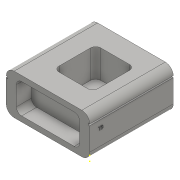
# Autodesk Inventor part: PassengerSectionNT
Saved by Autodesk Inventor 2016 (Build 200138000, 138)
## iProperties
Created: 2016-01-08
Part Number: PassengerSectionNT
Material: Generic
Document SubType Name: Modeling
Designer: 301278
Density: 1 g/cm^3
Appearance: Default
Author: 301278
Autodesk Inventor part; units mm, degrees
ref_plane "YZ Plane" through (0, 0, 0) normal (1, 0, 0) x (0, 1, 0)
ref_plane "XZ Plane" through (0, 0, 0) normal (0, 1, 0) x (-1, 0, 0)
ref_plane "XY Plane" through (0, 0, 0) normal (0, 0, 1) x (1, 0, 0)
sketch "Sketch1" plane through (0, 0, 0) normal (0, 0, 1) x (1, 0, 0)
  point P0 (0, 0)
sketch "Sketch2" plane through (0, 0, 0) normal (0, 0, 1) x (1, 0, 0)
  line L0 (7.62, 0) -> (72.898, 0)
  line L1 (80.518, 7.62) -> (80.518, 31.242)
  line L2 (72.898, 38.862) -> (7.62, 38.862)
  line L3 (0, 31.242) -> (0, 7.62)
  arc A0 (7.62, 38.862) -> (0, 31.242) centre (7.62, 31.242) ccw
  arc A1 (80.518, 31.242) -> (72.898, 38.862) centre (72.898, 31.242) ccw
  arc A2 (72.898, 0) -> (80.518, 7.62) centre (72.898, 7.62) ccw
  arc A3 (0, 7.62) -> (7.62, 0) centre (7.62, 7.62) ccw
  point P0 (0, 0)
  point P1 (80.518, 38.862)
  point P2 (80.518, 0)
  point P3 (0, 38.862)
  dimension "d0" = 80.518
  dimension "d1" = 38.862
  dimension "d2" = 7.62
  dimension "d3" = 7.62
  constraints: 8 end point, 8 point on circle, 8 point on line, 8 tangent, 4 centre point, 2 equal radius, 2 parallel, 1 horizontal, 1 perpendicular
  measures "d0" distance of point (0, 38.862) point (80.518, 38.862)
  measures "d1" distance of point (80.518, 38.862) point (80.518, 0)
  measures "d2" radius of A0
  measures "d3" radius of A1
extrude "Extrusion1" add sketch "Sketch2" along normal blind 80.518
sketch "Sketch3" plane through (0, 0, 80.518) normal (0, 0, 1) x (1, 0, 0)
  line L0 (13.716, 32.004) -> (66.802, 32.004)
  line L1 (71.882, 26.924) -> (71.882, 10.16)
  line L2 (66.802, 5.08) -> (13.716, 5.08)
  line L3 (8.636, 10.16) -> (8.636, 26.924)
  arc A0 (13.716, 32.004) -> (8.636, 26.924) centre (13.716, 26.924) ccw
  arc A1 (71.882, 26.924) -> (66.802, 32.004) centre (66.802, 26.924) ccw
  arc A2 (66.802, 5.08) -> (71.882, 10.16) centre (66.802, 10.16) ccw
  arc A3 (8.636, 10.16) -> (13.716, 5.08) centre (13.716, 10.16) ccw
  line L4 (72.898, 38.862) -> (7.62, 38.862) projected
  line L5 (0, 31.242) -> (0, 7.62) projected
  line L6 (80.518, 7.62) -> (80.518, 31.242) projected
  line L7 (72.898, 0) -> (7.62, 0) projected
  point P0 (0, 0)
  dimension "d6" = 5.08
  dimension "d7" = 5.08
  dimension "d8" = 6.858
  dimension "d9" = 8.636
  dimension "d10" = 8.636
  dimension "d11" = 5.08
  constraints: 8 end point, 8 point on circle, 8 tangent, 4 centre point, 2 equal radius, 2 parallel, 1 horizontal, 1 perpendicular
  measures "d6" radius of A0
  measures "d7" radius of A1
  measures "d8" distance between parallel lines of L4 L0
  measures "d9" distance between parallel lines of L5 L3
  measures "d10" distance between parallel lines of L6 L1
  measures "d11" distance from line of L7 L2.start
extrude "Extrusion2" cut sketch "Sketch3" against normal blind 14.478
sketch "Sketch4" plane through (0, 0, 0) normal (0, 0, -1) x (-1, 0, 0)
  line L0 (-65.659, 33.782) -> (-14.859, 33.782)
  line L1 (-9.779, 28.702) -> (-9.779, 10.16)
  line L2 (-14.859, 5.08) -> (-65.659, 5.08)
  line L3 (-70.739, 10.16) -> (-70.739, 28.702)
  arc A0 (-65.659, 33.782) -> (-70.739, 28.702) centre (-65.659, 28.702) ccw
  arc A1 (-70.739, 10.16) -> (-65.659, 5.08) centre (-65.659, 10.16) ccw
  arc A2 (-14.859, 5.08) -> (-9.779, 10.16) centre (-14.859, 10.16) ccw
  arc A3 (-9.779, 28.702) -> (-14.859, 33.782) centre (-14.859, 28.702) ccw
  line L4 (-7.62, 38.862) -> (-72.898, 38.862) projected
  line L5 (-72.898, 0) -> (-7.62, 0) projected
  line L6 (0, 7.62) -> (0, 31.242) projected
  line L7 (-80.518, 31.242) -> (-80.518, 7.62) projected
  point P0 (0, 0)
  dimension "d14" = 5.08
  dimension "d15" = 5.08
  dimension "d16" = 5.08
  dimension "d17" = 9.779
  dimension "d18" = 9.779
  constraints: 8 end point, 8 point on circle, 8 tangent, 4 centre point, 3 equal radius, 2 parallel, 1 horizontal, 1 perpendicular
  measures "d14" radius of A0
  measures "d15" distance between parallel lines of L4 L0
  measures "d16" distance between parallel lines of L5 L2
  measures "d17" distance between parallel lines of L6 L1
  measures "d18" distance between parallel lines of L7 L3
extrude "Extrusion3" cut sketch "Sketch4" against normal blind 14.478
sketch "Sketch5" plane through (14.859, 5.08, 0) normal (0, 1, 0) x (1, 0, 0)
  point P0 (-14.859, 0)
sketch "Sketch6" plane through (7.62, 38.862, 0) normal (0, 1, 0) x (1, 0, 0)
  line L0 (42.8172, -61.214) -> (15.357, -61.214)
  line L1 (10.277, -56.134) -> (10.277, -25.908)
  line L2 (15.357, -20.828) -> (42.8172, -20.828)
  line L3 (47.8972, -25.908) -> (47.8972, -56.134)
  arc A0 (42.8172, -61.214) -> (47.8972, -56.134) centre (42.8172, -56.134) ccw
  arc A1 (10.277, -56.134) -> (15.357, -61.214) centre (15.357, -56.134) ccw
  arc A2 (15.357, -20.828) -> (10.277, -25.908) centre (15.357, -25.908) ccw
  arc A3 (47.8972, -25.908) -> (42.8172, -20.828) centre (42.8172, -25.908) ccw
  line L4 (58.039, 0) -> (7.239, 0) projected
  point P0 (-7.62, 0)
  dimension "d21" = 5.08
  dimension "d22" = 40.386
  dimension "d23" = 20.828
  constraints: 8 end point, 8 point on circle, 8 tangent, 4 centre point, 3 equal radius, 2 parallel, 1 horizontal, 1 perpendicular
  measures "d21" radius of A0
  measures "d22" distance between parallel lines of L0 L2
  measures "d23" distance between parallel lines of L4 L2
extrude "Extrusion4" cut sketch "Sketch6" against normal blind 27.178
sketch "Sketch7" plane through (0, 7.62, 0) normal (-1, 0, 0) x (0, 0, 1)
  line L0 (8.0354, 16.9427) -> (12.7704, 16.9427) construction
  line L1 (12.7704, 16.9427) -> (12.7704, 13.7737) construction
  line L2 (12.7704, 13.7737) -> (8.0354, 13.7737) construction
  line L3 (8.0354, 13.7737) -> (8.0354, 16.9427) construction
  line L4 (9.0555, 13.833) -> (9.0555, 16.5204)
  line L5 (9.0555, 16.5204) -> (8.0329, 16.5204)
  line L6 (8.0329, 16.5204) -> (8.0329, 16.881)
  line L7 (8.0329, 16.881) -> (10.4832, 16.881)
  line L8 (10.4832, 16.881) -> (10.4832, 16.5204)
  line L9 (10.4832, 16.5204) -> (9.4606, 16.5204)
  line L10 (9.4606, 16.5204) -> (9.4606, 13.833)
  line L11 (9.4606, 13.833) -> (9.0555, 13.833)
  spline S0 degree 2 poles (10.6215, 15.8905) (10.6215, 16.1252) (10.7746, 16.5154) (10.908, 16.6562) knots 0 0 0 1 2 2 2
  spline S1 degree 2 poles (10.908, 16.6562) (11.034, 16.7921) (11.402, 16.9427) (11.5897, 16.9427) knots 0 0 0 1 2 2 2
  spline S2 degree 2 poles (11.5897, 16.9427) (11.7997, 16.9427) (12.1406, 16.8019) (12.2665, 16.6686) knots 0 0 0 1 2 2 2
  spline S3 degree 2 poles (12.2665, 16.6686) (12.4246, 16.5006) (12.5975, 15.9572) (12.5975, 15.5398) knots 0 0 0 1 2 2 2
  spline S4 degree 2 poles (12.5975, 15.5398) (12.5975, 15.1618) (12.4271, 14.4851) (12.2616, 14.2603) knots 0 0 0 1 2 2 2
  spline S5 degree 2 poles (12.2616, 14.2603) (12.0862, 14.0232) (11.5922, 13.7737) (11.2316, 13.7737) knots 0 0 0 1 2 2 2
  spline S6 degree 2 poles (11.2316, 13.7737) (11.1501, 13.7737) (10.9648, 13.791) (10.8858, 13.8157) knots 0 0 0 1 2 2 2
  line L12 (10.8858, 13.8157) -> (10.8858, 14.2084)
  line L13 (10.8858, 14.2084) -> (10.9055, 14.2084)
  spline S7 degree 2 poles (10.9055, 14.2084) (10.9574, 14.1788) (11.1748, 14.1269) (11.2859, 14.1269) knots 0 0 0 1 2 2 2
  spline S8 degree 2 poles (11.2859, 14.1269) (11.6861, 14.1269) (12.143, 14.6555) (12.1751, 15.1446) knots 0 0 0 1 2 2 2
  spline S9 degree 2 poles (12.1751, 15.1446) (12.0121, 15.0334) (11.7157, 14.9321) (11.5403, 14.9321) knots 0 0 0 1 2 2 2
  spline S10 degree 2 poles (11.5403, 14.9321) (11.3724, 14.9321) (11.0933, 15.0062) (10.9525, 15.1124) knots 0 0 0 1 2 2 2
  spline S11 degree 2 poles (10.9525, 15.1124) (10.7895, 15.2384) (10.6215, 15.6213) (10.6215, 15.8905) knots 0 0 0 1 2 2 2
  spline S12 degree 2 poles (12.185, 15.6311) (12.185, 15.9399) (12.0714, 16.3302) (11.9701, 16.4364) knots 0 0 0 1 2 2 2
  spline S13 degree 2 poles (11.9701, 16.4364) (11.8812, 16.5352) (11.696, 16.6093) (11.5873, 16.6093) knots 0 0 0 1 2 2 2
  spline S14 degree 2 poles (11.5873, 16.6093) (11.3353, 16.6093) (11.0365, 16.2487) (11.0365, 15.9078) knots 0 0 0 1 2 2 2
  spline S15 degree 2 poles (11.0365, 15.9078) (11.0365, 15.7151) (11.1353, 15.4657) (11.2439, 15.3767) knots 0 0 0 1 2 2 2
  spline S16 degree 2 poles (11.2439, 15.3767) (11.323, 15.3125) (11.5181, 15.2705) (11.6317, 15.2705) knots 0 0 0 1 2 2 2
  spline S17 degree 2 poles (11.6317, 15.2705) (11.7626, 15.2705) (12.064, 15.3619) (12.1776, 15.4385) knots 0 0 0 1 2 2 2
  spline S18 degree 2 poles (12.1776, 15.4385) (12.1801, 15.4681) (12.185, 15.5694) (12.185, 15.6311) knots 0 0 0 1 2 2 2
  point P0 (0, -7.62)
  constraints: 2 other
emboss "Emboss1" sketch "Sketch7" operation add depth 0.508 direction (1, 0, 0)
sketch "Sketch8" plane through (0, 0, 0) normal (0, 0, -1) x (-1, 0, 0)
  line L0 (0, 7.62) -> (0, 31.242) projected
  line L1 (0, 31.242) -> (-1.524, 31.242)
  line L2 (-1.524, 31.242) -> (-1.524, 29.718)
  line L3 (-1.524, 29.718) -> (0, 29.718)
  line L4 (0, 29.718) -> (0, 31.242)
  line L5 (-7.62, 38.862) -> (-72.898, 38.862) projected
  point P0 (0, 0)
  dimension "d28" = 7.62
  dimension "d29" = 1.524
  dimension "d30" = 1.524
  constraints: 8 end point, 2 parallel, 1 horizontal, 1 perpendicular, 1 point on line
  measures "d28" distance between parallel lines of L5 L1
  measures "d29" distance between parallel lines of L1 L3
  measures "d30" distance between parallel lines of L0 L2
extrude "Extrusion5" cut sketch "Sketch8" against normal blind 80.518
sketch "Sketch9" plane through (0, 0, 0) normal (0, 0, -1) x (-1, 0, 0)
  line L0 (-80.518, 7.62) -> (-80.518, 31.242) projected
  line L1 (-80.518, 31.242) -> (-78.994, 31.242)
  line L2 (-78.994, 31.242) -> (-78.994, 29.718)
  line L3 (-78.994, 29.718) -> (-80.518, 29.718)
  line L4 (-80.518, 29.718) -> (-80.518, 31.242)
  line L5 (-7.62, 38.862) -> (-72.898, 38.862) projected
  point P0 (0, 0)
  dimension "d33" = 1.524
  dimension "d34" = 1.524
  dimension "d35" = 7.62
  constraints: 8 end point, 2 parallel, 1 horizontal, 1 perpendicular, 1 point on line
  measures "d33" distance between parallel lines of L3 L1
  measures "d34" distance between parallel lines of L0 L2
  measures "d35" distance between parallel lines of L5 L1
extrude "Extrusion6" cut sketch "Sketch9" against normal blind 80.518
body "Solid1"
